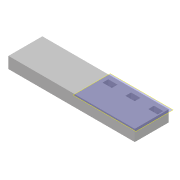
# Autodesk Inventor part: 10_Arm_Chip_xyz
Saved by Autodesk Inventor 2022 (Build 260153000, 153)
## iProperties
Created: 2023-01-22
Part Number: 10_Arm_Chip_xyz
Material: Generisch
Document SubType Name: Modeling
Designer: diederichbenedict
Density: 1 g/cm^3
Appearance: Vorgabe
Author: diederichbenedict
Autodesk Inventor part; units mm, degrees
ref_plane "YZ Plane" through (0, 0, 0) normal (1, 0, 0) x (0, 1, 0)
ref_plane "XZ Plane" through (0, 0, 0) normal (0, 1, 0) x (-1, 0, 0)
ref_plane "Arbeitsebene1" through (40, -32, 23.7) normal (0, -1, 0) x (-1, 0, 0)
sketch "Skizze1" plane through (40, -32, 23.7) normal (0, -1, 0) x (-1, 0, 0)
  line L0 (40, 23.7) -> (0, 23.7) projected
  line L1 (0, 0) -> (0, 23.7) projected
  line L2 (40, 0) -> (0, 0) projected
  line L3 (40, 0) -> (40, 23.7) projected
  line L4 (0, 23.7) -> (88.3, 23.7)
  line L5 (88.3, 23.7) -> (88.3, 0)
  line L6 (88.3, 0) -> (0, 0)
  line L7 (0, 0) -> (0, 23.7)
  line L8 (84.3, -24.675) -> (58.5, -24.675) projected
  line L9 (34.5, 23.7) -> (34.5, 29.7)
  line L10 (37.5, 23.7) -> (37.5, 29.7)
  line L11 (21.5, 23.7) -> (21.5, 29.7)
  line L12 (18.5, 23.7) -> (18.5, 29.7)
  line L13 (5.5, 23.7) -> (5.5, 29.7)
  line L14 (2.5, 23.7) -> (2.5, 29.7)
  line L15 (39.25, 20.7) -> (32.75, 20.7)
  line L16 (32.75, 20.7) -> (32.75, 16.7)
  line L17 (32.75, 16.7) -> (39.25, 16.7)
  line L18 (39.25, 16.7) -> (39.25, 20.7)
  line L19 (39.25, 20.7) -> (32.75, 16.7) construction
  line L20 (32.75, 20.7) -> (39.25, 16.7) construction
  line L21 (16.75, 20.7) -> (16.75, 16.7)
  line L22 (16.75, 16.7) -> (23.25, 16.7)
  line L23 (23.25, 16.7) -> (23.25, 20.7)
  line L24 (23.25, 20.7) -> (16.75, 16.7) construction
  line L25 (16.75, 20.7) -> (23.25, 16.7) construction
  line L26 (23.25, 20.7) -> (16.75, 20.7)
  line L27 (0.75, 20.7) -> (0.75, 16.7)
  line L28 (0.75, 16.7) -> (7.25, 16.7)
  line L29 (7.25, 16.7) -> (7.25, 20.7)
  line L30 (7.25, 20.7) -> (0.75, 16.7) construction
  line L31 (0.75, 20.7) -> (7.25, 16.7) construction
  line L32 (7.25, 20.7) -> (0.75, 20.7)
  circle A0 centre (12, 6.7) radius 1.4
  circle A1 centre (28, 6.7) radius 1.4
  point P0 (36, 18.7)
  point P1 (20, 18.7)
  point P2 (4, 18.7)
  dimension "d1" = 4
  dimension "d2" = 6.5
  dimension "d3" = 1.5
  dimension "d4" = 3
  dimension "d7" = 16
  dimension "d14" = 4
  dimension "d46" = 2.8
  dimension "d47" = 2.8
  dimension "d48" = 4.75
  dimension "d49" = 4.75
  dimension "d50" = 10
  dimension "d51" = 10
  constraints: 56 end point, 6 midpoint, 6 vertical, 4 parallel, 3 horizontal, 2 centre point, 2 perpendicular, 34 other
  measures "d1" distance of L16.end L15.end
  measures "d2" distance between parallel lines of L16 L18
  measures "d3" distance from line of point (36, 18.7) L10
  measures "d4" distance between parallel lines of L4 L15
  measures "d7" distance of L15.end L21.start
  measures "d14" horizontal distance of L5.end L8.start
  measures "d46" diameter of A0
  measures "d47" diameter of A1
  measures "d48" distance from line of A0.centre L29
  measures "d49" distance from line of A1.centre L23
  measures "d50" distance from line of A0.centre L22
  measures "d51" distance from line of A1.centre L22
ref_plane "Arbeitsebene2" through (0, -40, -6) normal (0, -1, 0) x (1, 0, 0)
extrude "Extrusion1" add sketch "Skizze1" along normal up to surface (8 mm away) contours L3 L2 L1 L0 | L4 L5 L6 L3 | A0 | A1
sketch "Skizze3" plane through (-48.3, -40, 0) normal (0, -1, 0) x (1, 0, 0)
  line L0 (29.8, 56.375) -> (4, 56.375)
  line L1 (4, 56.375) -> (4, 52.375)
  line L2 (29.8, 52.375) -> (4, 52.375)
  line L3 (29.8, 56.375) -> (29.8, 52.375)
  line L4 (49.05, 3) -> (55.55, 3) projected
  line L5 (49.05, 7) -> (49.05, 3) projected
  line L6 (55.55, 7) -> (49.05, 7) projected
  line L7 (55.55, 3) -> (55.55, 7) projected
  line L8 (71.55, 3) -> (71.55, 7) projected
  line L9 (65.05, 3) -> (71.55, 3) projected
  line L10 (65.05, 7) -> (65.05, 3) projected
  line L11 (71.55, 7) -> (65.05, 7) projected
  line L12 (87.55, 3) -> (87.55, 7) projected
  line L13 (81.05, 3) -> (87.55, 3) projected
  line L14 (81.05, 7) -> (81.05, 3) projected
  line L15 (87.55, 7) -> (81.05, 7) projected
  line L16 (0, 0) -> (0, 23.7) projected
  line L17 (88.3, 0) -> (0, 0) projected
  line L18 (88.3, 23.7) -> (88.3, 0) projected
  line L19 (0, 23.7) -> (88.3, 23.7) projected
  line L20 (0, 23.7) -> (27, 23.7)
  line L21 (27, 23.7) -> (27, 59.7)
  line L22 (27, 59.7) -> (0, 59.7)
  line L23 (0, 59.7) -> (0, 23.7)
  line L24 (3.8, 52.175) -> (3.8, 56.575)
  line L25 (3.8, 56.575) -> (30, 56.575)
  line L26 (30, 56.575) -> (30, 52.175)
  line L27 (30, 52.175) -> (3.8, 52.175)
  arc A0 (0, 59.7) -> (0, 46.9788) centre (0, 53.3394) ccw
  point P0 (48.3, 0)
  point P1 (27, 52.175)
  point P2 (27, 56.575)
  dimension "d22" = 36
  dimension "d23" = 27
  dimension "d24" = 0.2
  constraints: 24 end point, 5 point on line, 2 parallel, 2 point on circle, 1 centre point, 1 horizontal, 1 perpendicular, 1 tangent, 3 other
  measures "d22" distance between parallel lines of L19 L22
  measures "d23" distance between parallel lines of L23 L21
  measures "d24" distance between parallel lines of L2 L27
extrude "Extrusion2" add sketch "Skizze3" against normal up to surface (8 mm away) contours L25 L24 L27 L21 L19 L23 L22 | L23 A0
chamfer "Fase1" distance 10 angle 45 1 edges at (-21.3, -36, 23.7)
sketch "Skizze4" plane through (-48.3, -40, 0) normal (0, -1, 0) x (1, 0, 0)
  line L0 (49.05, 3) -> (55.55, 3) projected
  line L1 (49.05, 7) -> (49.05, 3) projected
  line L2 (55.55, 7) -> (49.05, 7) projected
  line L3 (55.55, 3) -> (55.55, 7) projected
  line L4 (71.55, 3) -> (71.55, 7) projected
  line L5 (65.05, 3) -> (71.55, 3) projected
  line L6 (65.05, 7) -> (65.05, 3) projected
  line L7 (71.55, 7) -> (65.05, 7) projected
  line L8 (87.55, 3) -> (87.55, 7) projected
  line L9 (81.05, 3) -> (87.55, 3) projected
  line L10 (81.05, 7) -> (81.05, 3) projected
  line L11 (87.55, 7) -> (81.05, 7) projected
  line L12 (0, 0) -> (0, 46.9788) projected
  line L13 (88.3, 0) -> (0, 0) projected
  line L14 (88.3, 23.7) -> (88.3, 0) projected
  line L15 (37, 23.7) -> (88.3, 23.7) projected
  line L16 (27, 33.7) -> (37, 23.7) projected
  line L17 (27, 33.7) -> (27, 52.175) projected
  line L18 (27, 52.175) -> (3.8, 52.175) projected
  line L19 (3.8, 52.175) -> (3.8, 56.575) projected
  line L20 (3.8, 56.575) -> (27, 56.575) projected
  line L21 (27, 56.575) -> (27, 59.7) projected
  line L22 (27, 59.7) -> (0, 59.7) projected
  arc A0 (0, 59.7) -> (0, 46.9788) centre (0, 53.3394) ccw projected
  line L23 (0, 0) -> (0, 46.9788) projected
  line L24 (0, 46.9788) -> (27, 46.9788)
  line L25 (27, 33.7) -> (27, 52.175) projected
  point P0 (48.3, 0)
  constraints: 2 end point, 1 perpendicular, 1 point on line
extrude "Extrusion3" add sketch "Skizze4" along normal blind 20 contours A0 L22 L21 L20 L19 L18 L17 L24
ref_plane "Arbeitsebene3" through (-32.3, -40, 0) normal (-1, 0, 0) x (0, 0, 1)
sketch "Skizze5" plane through (-32.3, -40, 0) normal (-1, 0, 0) x (0, 0, 1)
  line L0 (0, 0) -> (46.9788, 0) projected
  line L1 (46.9788, 0) -> (46.9788, -20) projected
  line L2 (46.9788, 0) -> (46.9788, -20) projected
  line L3 (46.9788, -20) -> (26.9788, 0)
  line L4 (33.7, 0) -> (23.7, 0) projected
  line L5 (46.9788, -20) -> (75.2631, -20) construction
  line L6 (26.9788, 0) -> (46.9788, 0)
  point P0 (0, 40)
  point P1 (26.9788, 0)
  dimension "d33" = 135
  constraints: 6 end point, 1 equal length, 1 horizontal, 1 perpendicular, 1 point on line
  measures "d33" angle of L5 L3
extrude "Extrusion4" add sketch "Skizze5" along normal mid plane 22
ref_plane "Arbeitsebene4" through (-48.3, -60, 26.9788) normal (0, 0, -1) x (-1, 0, 0)
sketch "Skizze6" plane through (-48.3, -60, 26.9788) normal (0, 0, -1) x (-1, 0, 0)
  line L0 (-5, 0) -> (-27, 0) projected
  line L1 (-5, 20) -> (-5, 0) projected
  line L2 (-27, 20) -> (-5, 20) projected
  line L3 (-27, 0) -> (-27, 20) projected
  circle A0 centre (-16, 5.2138) radius 1.4
  circle A1 centre (-16, 15.5099) radius 1.4
  point P0 (-48.3, 60)
  dimension "d37" = 2.8
  dimension "d38" = 2.8
  constraints: 2 centre point
  measures "d37" diameter of A0
  measures "d38" diameter of A1
hole "Bohrung2" at (-32.3, -54.7862, 26.9788) at (-32.3, -44.4901, 26.9788) direction (0, 0, 1) diameter 2.8 depth 22 tip angle 118 counterbore diameter 6.5 counterbore depth 17
chamfer "Fase2" distance 2 angle 45 3 edges at (-29.3203, -53.4886, 40.4674) (-35.2797, -53.4886, 40.4674) (-32.3, -47.7401, 34.7189)
sketch "Skizze7" plane through (-48.3, -40, 0) normal (0, -1, 0) x (1, 0, 0)
  line L0 (48.3, -6) -> (48.3, 0) projected
  line L1 (88.3, -6) -> (48.3, -6) projected
  line L2 (88.3, -6.15) -> (33.3, -6.15)
  line L3 (33.3, -6.15) -> (33.3, -13.15)
  line L4 (33.3, -13.15) -> (88.3, -13.15)
  line L5 (88.3, -13.15) -> (88.3, -6.15)
  line L6 (88.3, 0) -> (0, 0) projected
  line L7 (0, 0) -> (48, 0)
  line L8 (48, 0) -> (48, -6.15)
  line L9 (48, -6.15) -> (0, -6.15)
  line L10 (0, -6.15) -> (0, 0)
  point P0 (48, 0)
  dimension "d55" = 55
  dimension "d56" = 7
  dimension "d57" = 0.15
  dimension "d58" = 0.3
  constraints: 16 end point, 4 parallel, 2 horizontal, 2 perpendicular, 1 point on line
  measures "d55" distance of L4.end L3.end
  measures "d56" distance of L3.end L2.end
  measures "d57" distance between parallel lines of L2 L1
  measures "d58" distance between parallel lines of L8 L0
extrude "Extrusion5" add sketch "Skizze7" against normal up to surface (8 mm away)
sketch "Skizze8" plane through (40, -40, 0) normal (0, -1, 0) x (1, 0, 0)
  line L0 (-83.3, 26.9788) -> (-83.3, 46.9788) projected
  line L1 (-83.3, 46.9788) -> (-88.3, 46.9788) projected
  line L2 (-88.3, -6.15) -> (-88.3, 46.9788) projected
  line L3 (-88.3, -6.15) -> (-55, -6.15) projected
  line L4 (-55, -6.15) -> (-55, -13.15) projected
  line L5 (-55, -13.15) -> (0, -13.15) projected
  line L6 (0, -13.15) -> (0, -6.15) projected
  line L7 (0, -6.15) -> (-40.3, -6.15) projected
  line L8 (-40.3, -6.15) -> (-40.3, 0) projected
  line L9 (0, 0) -> (-40.3, 0) projected
  line L10 (0, 23.7) -> (0, 0) projected
  line L11 (-51.3, 23.7) -> (0, 23.7) projected
  line L12 (-61.3, 33.7) -> (-51.3, 23.7) projected
  line L13 (-61.3, 33.7) -> (-61.3, 26.9788) projected
  line L14 (-61.3, 26.9788) -> (-70.8603, 26.9788) projected
  line L15 (-73.7397, 26.9788) -> (-83.3, 26.9788) projected
  line L16 (-0.75, 3) -> (-0.75, 7) projected
  line L17 (-7.25, 3) -> (-0.75, 3) projected
  line L18 (-7.25, 7) -> (-7.25, 3) projected
  line L19 (-0.75, 7) -> (-7.25, 7) projected
  line L20 (-16.75, 3) -> (-16.75, 7) projected
  line L21 (-23.25, 3) -> (-16.75, 3) projected
  line L22 (-23.25, 7) -> (-23.25, 3) projected
  line L23 (-16.75, 7) -> (-23.25, 7) projected
  line L24 (-39.25, 3) -> (-32.75, 3) projected
  line L25 (-39.25, 7) -> (-39.25, 3) projected
  line L26 (-32.75, 7) -> (-39.25, 7) projected
  line L27 (-32.75, 3) -> (-32.75, 7) projected
  line L28 (0, 23.7) -> (-51.3, 23.7) projected
  line L29 (0, 23.7) -> (-30.5, 23.7)
  line L30 (-30.5, 23.7) -> (-30.5, 0)
  line L31 (-30.5, 0) -> (0, 0)
  line L32 (0, 0) -> (0, 23.7)
  line L33 (-30.5, 23.7) -> (-40.3, 23.7)
  line L34 (-40.3, 23.7) -> (-40.3, 13.7)
  line L35 (-40.3, 13.7) -> (-30.5, 13.7)
  line L36 (-30.5, 13.7) -> (-30.5, 23.7)
  point P0 (-40, 0)
  point P1 (-30.5, 13.7)
  dimension "d61" = 30.5
  dimension "d62" = 10
  constraints: 16 end point, 4 parallel, 2 horizontal, 2 perpendicular, 1 horizontal alignment, 1 point on line
  measures "d61" distance of L31.end L30.end
  measures "d62" distance of L34.end L33.end
extrude "Extrusion6" cut sketch "Skizze8" against normal blind 10 contours L9 L30 L11 L10 | L35 L34 L11 L30 | L17 L18 L19 L16 | L21 L22 L23 L20
sketch "Skizze9" plane through (40, -40, -13.15) normal (0, 0, -1) x (-1, 0, 0)
  circle A0 centre (4, 5.5) radius 1.5
  circle A1 centre (20, 5.5) radius 1.5
  circle A2 centre (36, 5.5) radius 1.5
  circle A3 centre (36, 5.4751) radius 1.5
  line L0 (40.3, 8) -> (30.5, 8) projected
  point P0 (40, 40)
  dimension "d70" = 2.5
  dimension "d71" = 2.5
  dimension "d72" = 2.5
  constraints: 4 centre point
  measures "d70" distance from line of A2.centre L0
  measures "d71" distance from line of A1.centre L0
  measures "d72" distance from line of L0 A0.centre
extrude "Extrusion7" cut sketch "Skizze9" against normal through all contours A0 | A1 | A2 A3 | A3 A2 picked at (36.0536, 4.9955) picked at (36.0536, 6.981)
chamfer "Fase3" distance 2 angle 45 4 edges at (-15, -36, -13.15) (-48.3, -36, -6.15) (-15, -36, -6.15) (-0.3, -36, 23.7)
sketch "Skizze10" plane through (-48.3, -40, 46.9788) normal (0, -1, 0) x (1, 0, 0)
  line L0 (46, -23.2788) -> (48, -25.2788) projected
  line L1 (37, -23.2788) -> (46, -23.2788) projected
  line L2 (27, -13.2788) -> (37, -23.2788) projected
  line L3 (27, -13.2788) -> (27, -20) projected
  line L4 (27, -20) -> (17.4397, -20) projected
  line L5 (14.5603, -20) -> (5, -20) projected
  line L6 (5, -20) -> (5, 0) projected
  line L7 (5, 0) -> (0, 0) projected
  line L8 (0, -51.1288) -> (0, 0) projected
  line L9 (2, -53.1288) -> (0, -51.1288) projected
  line L10 (2, -53.1288) -> (31.3, -53.1288) projected
  line L11 (33.3, -55.1288) -> (31.3, -53.1288) projected
  line L12 (33.3, -55.1288) -> (33.3, -58.1288) projected
  line L13 (35.3, -60.1288) -> (33.3, -58.1288) projected
  line L14 (35.3, -60.1288) -> (88.3, -60.1288) projected
  line L15 (88.3, -60.1288) -> (88.3, -53.1288) projected
  line L16 (88.3, -53.1288) -> (48, -53.1288) projected
  line L17 (48, -53.1288) -> (48, -46.9788) projected
  line L18 (57.8, -46.9788) -> (48, -46.9788) projected
  line L19 (57.8, -46.9788) -> (57.8, -33.2788) projected
  line L20 (57.8, -33.2788) -> (48, -33.2788) projected
  line L21 (48, -33.2788) -> (48, -25.2788) projected
  line L22 (49.05, -43.9788) -> (55.55, -43.9788) projected
  line L23 (49.05, -39.9788) -> (49.05, -43.9788) projected
  line L24 (55.55, -39.9788) -> (49.05, -39.9788) projected
  line L25 (55.55, -43.9788) -> (55.55, -39.9788) projected
  point P0 (48.3, -46.9788)
  constraints: 1 horizontal alignment
